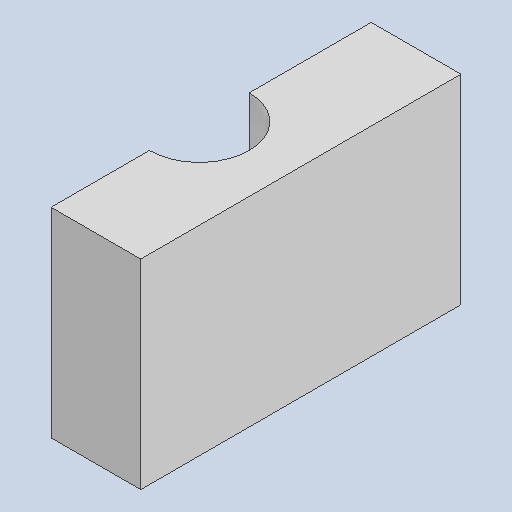
# Autodesk Inventor part: test1
Saved by Autodesk Inventor 2025 (Build 290162000, 162)
## iProperties
Created: 2025-04-20
Part Number: test1
Material: Generic
Document SubType Name: Sheet Metal
Designer: Pravoslav
Density: 1 g/cm^3
Sheet Metal Rule: Default_mm
Appearance: Default
Author: Pravoslav
Autodesk Inventor part; units mm, degrees
ref_plane "YZ Plane" through (0, 0, 0) normal (1, 0, 0) x (0, 1, 0)
ref_plane "XZ Plane" through (0, 0, 0) normal (0, 1, 0) x (-1, 0, 0)
ref_plane "XY Plane" through (0, 0, 0) normal (0, 0, 1) x (1, 0, 0)
sketch "Sketch1" plane through (0, 0, 0) normal (0, 1, 0) x (-1, 0, 0)
  line L0 (0, 1.6745) -> (-1.7969, 1.6745)
  line L1 (-1.7969, 1.6745) -> (-1.7969, -4.7401)
  line L2 (-1.7969, -4.7401) -> (0, -4.7401)
  line L3 (0, -4.7401) -> (0, 1.6745)
  circle A0 centre (0, -1.2958) radius 1
  point P0 (0, 0)
  point P1 (0, -2.2958)
  point P2 (0, -0.2958)
  dimension "d0" = 2
  constraints: 8 end point, 2 parallel, 1 centre point, 1 horizontal, 1 perpendicular, 1 point on line
  measures "d0" diameter of A0
extrude "Extrusion1" add sketch "Sketch1" along normal blind 4 contours L3 A0 L2 L1 L0
equation "\"BendRadius\" = Thickness"
equation "\"BendReliefWidth\" = Thickness"
equation "\"BendReliefDepth\" = 0.5 * Thickness"
equation "\"CornerReliefSize\" = 4 * Thickness"
equation "\"MinimumRemnant\" = 2 * Thickness"
equation "\"TransitionRadius\" = BendRadius"
equation "\"JacobiRadiusSize\" = BendRadius"
equation "\"GapSize\" = Thickness"
equation "\"Thickness\" = 0.5"
body "Solid1"
